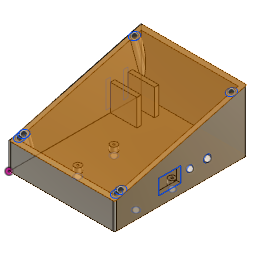
RotCase v3 (Autodesk Fusion 360 design; units mm, degrees)
Autodesk Fusion 360 part; units mm, degrees
note: some values were not read from the file. Set by a fixed rule: which face or edge a step refers to.
sketch "Sketch1" plane through (0, 0, 0) normal (1, 0, 0) x (0, 1, 0)
  line L0 (0, 0) -> (150, 0)
  line L1 (150, 0) -> (150, 70)
  line L2 (0, 0) -> (0, 30)
  line L3 (0, 30) -> (150, 70)
  line L4 (135, 5) -> (130, 5)
  line L5 (130, 5) -> (130, 35)
  line L6 (130, 35) -> (135, 35)
  line L7 (135, 35) -> (135, 5)
  line L8 (115, 5) -> (110, 5)
  line L9 (110, 5) -> (110, 35)
  line L10 (110, 35) -> (115, 35)
  line L11 (115, 35) -> (115, 5)
  dimension "d1" = 150
  dimension "d2" = 70
  dimension "d3" = 30
  constraint coincident L0.start L2.start
  constraint horizontal L0
  constraint perpendicular L0 L1
  constraint perpendicular L0 L2
  constraint horizontal L4
  constraint vertical L5
  constraint horizontal L6
  constraint vertical L7
  constraint horizontal L8
  constraint vertical L9
  constraint horizontal L10
  constraint vertical L11
  measures "d1" distance of L0.start L0.end
  measures "d2" distance of L0.end L1.end
  measures "d3" distance of L0.start L2.end
extrude "Extrude1" add sketch "Sketch1" along normal blind 120 contours L0 L1 L2 L3 | L4 L5 L6 L7 | L8 L9 L10 L11
shell "Shell1" thickness 5 removed faces 1 at (80, 50, 43.3333)
sketch "Sketch2" plane through (0, -7.4689, 28.0083) normal (0, -0.257663, 0.966235) x (1, 0, 0)
  line L0 (5, 157.7969) -> (115, 157.7969)
  line L1 (115, 157.7969) -> (115, 12.9046)
  line L2 (115, 12.9046) -> (5, 12.9046)
  line L3 (5, 12.9046) -> (5, 157.7969)
  line L4 (0, 162.9716) -> (0, 7.7299)
  line L5 (0, 7.7299) -> (120, 7.7299)
  line L6 (120, 7.7299) -> (120, 162.9716)
  line L7 (120, 162.9716) -> (0, 162.9716)
  circle A0 centre (115, 149.8964) radius 5
  circle A1 centre (5, 150) radius 5
  circle A2 centre (5, 15.0104) radius 5
  circle A3 centre (115, 14.9807) radius 5
  dimension "d7" = 10
  dimension "d8" = 10
  dimension "d9" = 10
  dimension "d10" = 10
  constraint coincident L1 A0.centre
  constraint coincident L3 A1.centre
  constraint coincident L3 A2.centre
  constraint coincident L1 A3.centre
  measures "d7" diameter of A0
  measures "d8" diameter of A1
  measures "d9" diameter of A2
  measures "d10" diameter of A3
extrude "Extrude2" add sketch "Sketch2" along normal up to surface contours L1 A0 picked at (113.338, 150.021) end surface through (0, 145, 0) normal (0, -1, 0) offset 0
sketch "Sketch3" plane through (0, -7.4689, 28.0083) normal (0, -0.257663, 0.966235) x (1, 0, 0)
  line L0 (5, 157.7969) -> (115, 157.7969)
  line L1 (115, 157.7969) -> (115, 154.8964)
  arc A0 (115, 154.8964) -> (115, 144.8964) centre (115, 149.8964) ccw
  line L2 (115, 144.8964) -> (115, 12.9046)
  line L3 (115, 12.9046) -> (5, 12.9046)
  line L4 (5, 12.9046) -> (5, 157.7969)
  line L5 (0, 162.9716) -> (0, 7.7299)
  line L6 (0, 7.7299) -> (120, 7.7299)
  line L7 (120, 7.7299) -> (120, 162.9716)
  line L8 (120, 162.9716) -> (0, 162.9716)
  circle A1 centre (5, 150) radius 5
  dimension "d13" = 10
  constraint coincident L4 A1.centre
  measures "d13" diameter of A1
extrude "Extrude3" add sketch "Sketch3" along normal up to surface contours L4 A1 picked at (6.9904, 150.6924) end surface through (0, 145, 0) normal (0, -1, 0) offset 0
sketch "Sketch4" plane through (0, -7.4689, 28.0083) normal (0, -0.257663, 0.966235) x (1, 0, 0)
  line L0 (5, 157.7969) -> (115, 157.7969)
  line L1 (115, 157.7969) -> (115, 154.8964)
  arc A0 (115, 154.8964) -> (115, 144.8964) centre (115, 149.8964) ccw
  line L2 (115, 144.8964) -> (115, 12.9046)
  line L3 (115, 12.9046) -> (5, 12.9046)
  line L4 (5, 12.9046) -> (5, 145)
  arc A1 (5, 145) -> (5, 155) centre (5, 150) ccw
  line L5 (5, 155) -> (5, 157.7969)
  line L6 (0, 162.9716) -> (0, 7.7299)
  line L7 (0, 7.7299) -> (120, 7.7299)
  line L8 (120, 7.7299) -> (120, 162.9716)
  line L9 (120, 162.9716) -> (0, 162.9716)
  circle A2 centre (115, 20) radius 5
  circle A3 centre (5, 20) radius 5
  dimension "d16" = 10
  dimension "d17" = 10
  constraint coincident L2 A2.centre
  constraint coincident L4 A3.centre
  measures "d16" diameter of A2
  measures "d17" diameter of A3
extrude "Extrude4" add sketch "Sketch4" along normal up to surface contours L4 A3 | L2 A2 picked at (6.3706, 18.5304) picked at (113.338, 19.8754) end surface through (0, 0, 5) normal (0, 0, 1) offset 0
sketch "Sketch5" plane through (0, -7.4689, 28.0083) normal (0, -0.257663, 0.966235) x (1, 0, 0)
  line L0 (5, 157.7969) -> (115, 157.7969)
  line L1 (115, 157.7969) -> (115, 154.8964)
  arc A0 (115, 154.8964) -> (115, 144.8964) centre (115, 149.8964) ccw
  line L2 (115, 144.8964) -> (115, 25)
  arc A1 (115, 25) -> (115, 15) centre (115, 20) ccw
  line L3 (115, 15) -> (115, 12.9046)
  line L4 (115, 12.9046) -> (5, 12.9046)
  line L5 (5, 12.9046) -> (5, 15)
  arc A2 (5, 15) -> (5, 25) centre (5, 20) ccw
  line L6 (5, 25) -> (5, 145)
  arc A3 (5, 145) -> (5, 155) centre (5, 150) ccw
  line L7 (5, 155) -> (5, 157.7969)
  line L8 (0, 162.9716) -> (0, 7.7299)
  line L9 (0, 7.7299) -> (120, 7.7299)
  line L10 (120, 7.7299) -> (120, 162.9716)
  line L11 (120, 162.9716) -> (0, 162.9716)
hole "Hole1" at (115, 137.3663, 66.631) direction (0, 0.257663, -0.966235) diameter 1.8 depth 20 tip angle 118
hole "Hole2" at (5, 137.4664, 66.6577) direction (0, 0.257663, -0.966235) diameter 2 depth 22 tip angle 118
sketch "Sketch6" plane through (0, -7.4689, 28.0083) normal (0, -0.257663, 0.966235) x (1, 0, 0)
  circle A0 centre (5, 150) radius 1
  circle A1 centre (115, 149.8964) radius 0.9
  line L0 (5, 157.7969) -> (115, 157.7969)
  line L1 (115, 157.7969) -> (115, 154.8964)
  arc A2 (115, 154.8964) -> (115, 144.8964) centre (115, 149.8964) ccw
  line L2 (115, 144.8964) -> (115, 25)
  arc A3 (115, 25) -> (115, 15) centre (115, 20) ccw
  line L3 (115, 15) -> (115, 12.9046)
  line L4 (115, 12.9046) -> (5, 12.9046)
  line L5 (5, 12.9046) -> (5, 15)
  arc A4 (5, 15) -> (5, 25) centre (5, 20) ccw
  line L6 (5, 25) -> (5, 145)
  arc A5 (5, 145) -> (5, 155) centre (5, 150) ccw
  line L7 (5, 155) -> (5, 157.7969)
  line L8 (0, 162.9716) -> (0, 7.7299)
  line L9 (0, 7.7299) -> (120, 7.7299)
  line L10 (120, 7.7299) -> (120, 162.9716)
  line L11 (120, 162.9716) -> (0, 162.9716)
hole "Hole3" at (115, 11.8558, 33.1616) direction (0, 0.257663, -0.966235) diameter 2 depth 22 tip angle 118
sketch "Sketch7" plane through (0, -7.4689, 28.0083) normal (0, -0.257663, 0.966235) x (1, 0, 0)
  circle A0 centre (115, 20) radius 1
  circle A1 centre (5, 150) radius 1
  circle A2 centre (115, 149.8964) radius 0.9
  line L0 (5, 157.7969) -> (115, 157.7969)
  line L1 (115, 157.7969) -> (115, 154.8964)
  arc A3 (115, 154.8964) -> (115, 144.8964) centre (115, 149.8964) ccw
  line L2 (115, 144.8964) -> (115, 25)
  arc A4 (115, 25) -> (115, 15) centre (115, 20) ccw
  line L3 (115, 15) -> (115, 12.9046)
  line L4 (115, 12.9046) -> (5, 12.9046)
  line L5 (5, 12.9046) -> (5, 15)
  arc A5 (5, 15) -> (5, 25) centre (5, 20) ccw
  line L6 (5, 25) -> (5, 145)
  arc A6 (5, 145) -> (5, 155) centre (5, 150) ccw
  line L7 (5, 155) -> (5, 157.7969)
  line L8 (0, 162.9716) -> (0, 7.7299)
  line L9 (0, 7.7299) -> (120, 7.7299)
  line L10 (120, 7.7299) -> (120, 162.9716)
  line L11 (120, 162.9716) -> (0, 162.9716)
hole "Hole4" at (5, 11.8558, 33.1616) direction (0, 0.257663, -0.966235) diameter 2 depth 22 tip angle 118
fillet "Fillet1" radius 2 4 edges at (0, 150, 35) (120, 150, 35) (120, 0, 15) (0, 0, 15)
sketch "Sketch8" plane through (120, 0, 0) normal (1, 0, 0) x (0, 1, 0)
  line L0 (2, 30.5333) -> (2, 0)
  line L1 (2, 0) -> (148, 0)
  line L2 (148, 0) -> (148, 69.4667)
  line L3 (148, 69.4667) -> (2, 30.5333)
sketch "Sketch9" plane through (120, 0, 0) normal (1, 0, 0) x (0, 1, 0)
  line L0 (50, 11) -> (75, 11)
  line L1 (75, 11) -> (75, 28)
  line L2 (75, 28) -> (50, 28)
  line L3 (50, 28) -> (50, 11)
  dimension "d33" = 17
  dimension "d34" = 25
  constraint horizontal L0
  constraint vertical L1
  constraint horizontal L2
  constraint vertical L3
  measures "d33" distance of L0.start L2.end
  measures "d34" distance of L0.start L0.end
extrude "Extrude5" cut sketch "Sketch9" against normal up to surface (5 mm away)
sketch "Sketch10" plane through (120, 0, 0) normal (1, 0, 0) x (0, 1, 0)
  circle A0 centre (85, 20) radius 3.25
  circle A1 centre (105, 20) radius 4
  dimension "d37" = 6.5
  dimension "d38" = 8
  measures "d37" diameter of A0
  measures "d38" diameter of A1
extrude "Extrude6" cut sketch "Sketch10" against normal up to surface (5 mm away)
sketch "Sketch11" plane through (0, -7.4689, 28.0083) normal (0, -0.257663, 0.966235) x (1, 0, 0)
  circle A0 centre (5, 20) radius 1
  circle A1 centre (115, 20) radius 1
  circle A2 centre (5, 150) radius 1
  circle A3 centre (115, 149.8964) radius 0.9
  line L0 (5, 157.7969) -> (115, 157.7969)
  line L1 (115, 157.7969) -> (115, 154.8964)
  arc A4 (115, 154.8964) -> (115, 144.8964) centre (115, 149.8964) ccw
  line L2 (115, 144.8964) -> (115, 25)
  arc A5 (115, 25) -> (115, 15) centre (115, 20) ccw
  line L3 (115, 15) -> (115, 12.9046)
  line L4 (115, 12.9046) -> (5, 12.9046)
  line L5 (5, 12.9046) -> (5, 15)
  arc A6 (5, 15) -> (5, 25) centre (5, 20) ccw
  line L6 (5, 25) -> (5, 145)
  arc A7 (5, 145) -> (5, 155) centre (5, 150) ccw
  line L7 (5, 155) -> (5, 157.7969)
  ellipse E0 centre (2, 9.7998) end of major axis (2, 7.7299) minor radius 2 (0, 9.7998) -> (2, 7.7299) ccw
  line L8 (2, 7.7299) -> (118, 7.7299)
  ellipse E1 centre (118, 9.7998) end of major axis (118, 7.7299) minor radius 2 (118, 7.7299) -> (120, 9.7998) ccw
  line L9 (120, 9.7998) -> (120, 160.9017)
  ellipse E2 centre (118, 160.9017) end of major axis (118, 162.9716) minor radius 2 (120, 160.9017) -> (118, 162.9716) ccw
  line L10 (118, 162.9716) -> (2, 162.9716)
  ellipse E3 centre (2, 160.9017) end of major axis (2, 162.9716) minor radius 2 (2, 162.9716) -> (0, 160.9017) ccw
  line L11 (0, 160.9017) -> (0, 9.7998)
sketch "Sketch12" plane through (60, 75, 50) normal (0, -0.257663, 0.966235) x (1, 0, 0)
sketch "Sketch13" plane through (0, 0, 0) normal (0, 0, 1) x (1, 0, 0)
sketch "Sketch14" plane through (0, -7.4689, 28.0083) normal (0, -0.257663, 0.966235) x (1, 0, 0)
sketch "Sketch15" plane through (0, 0, 0) normal (0, 0, -1) x (1, 0, 0)
  arc A0 (2, 0) -> (0, -2) centre (2, -2) ccw
  line L0 (0, -2) -> (0, -148)
  arc A1 (0, -148) -> (2, -150) centre (2, -148) ccw
  line L1 (2, -150) -> (118, -150)
  arc A2 (118, -150) -> (120, -148) centre (118, -148) ccw
  line L2 (120, -148) -> (120, -2)
  arc A3 (120, -2) -> (118, 0) centre (118, -2) ccw
  line L3 (118, 0) -> (2, 0)
  circle A4 centre (110.1015, -75) radius 4
  circle A5 centre (44.1015, -75) radius 4
  circle A6 centre (110.1015, -34) radius 4
  circle A7 centre (44.1015, -34) radius 4
  dimension "d42" = 8
  dimension "d45" = -66
  dimension "d46" = 41
  measures "d42" diameter of A4
extrude "Extrude7" add sketch "Sketch15" against normal blind 11 contours A4 | A5 | A6 | A7
sketch "Sketch16" plane through (0, 0, 0) normal (0, 0, -1) x (1, 0, 0)
  arc A0 (2, 0) -> (0, -2) centre (2, -2) ccw
  line L0 (0, -2) -> (0, -148)
  arc A1 (0, -148) -> (2, -150) centre (2, -148) ccw
  line L1 (2, -150) -> (118, -150)
  arc A2 (118, -150) -> (120, -148) centre (118, -148) ccw
  line L2 (120, -148) -> (120, -2)
  arc A3 (120, -2) -> (118, 0) centre (118, -2) ccw
  line L3 (118, 0) -> (2, 0)
hole "Hole7" at (110.1015, 34, 0) direction (0, 0, 1) diameter 2.2 depth 11 tip angle 180 counterbore diameter 2.6 counterbore depth 1
pattern_linear "R-Pattern1" count 2 spacing 66 along (-1, 0, 0) count 2 spacing 41 along (0, 1, 0) of "Hole7"
extrude "Extrude9" add sketch "Sketch1" along normal blind 35 contours L4 L5 L6 L7 | L8 L9 L10 L11
